Autodesk Fusion 360 part; units mm, degrees
(part 2 of 2)
sketch "Skizze5" plane through (29.2112, 25.4006, 12) normal (0, 0, 1) x (1, 0, 0)
  line L0 (-31.25, 31.4) -> (31.25, 31.4)
  arc A0 (-31.25, 31.4) -> (-34.25, 28.4) centre (-31.25, 28.4) ccw
  line L1 (-34.25, -25.4) -> (-34.25, 28.4)
  line L2 (-32.25, -25.4) -> (-32.25, 28.4)
  arc A1 (-31.25, 29.4) -> (-32.25, 28.4) centre (-31.25, 28.4) ccw
  line L3 (-31.25, 29.4) -> (31.25, 29.4)
  arc A2 (32.25, 28.4) -> (31.25, 29.4) centre (31.25, 28.4) ccw
  line L4 (32.25, 28.4) -> (32.25, -25.4)
  arc A3 (34.25, 28.4) -> (31.25, 31.4) centre (31.25, 28.4) ccw
  line L5 (34.25, 28.4) -> (34.25, -25.4)
  line L6 (34.25, -25.4) -> (-34.25, -25.4)
  line L7 (-32.25, -15.7) -> (32.25, -15.7)
  line L8 (-32.25, -13.7) -> (32.25, -13.7)
  line L9 (-33.05, -25.4) -> (-33.05, 28.4)
  arc A4 (-31.25, 30.2) -> (-33.05, 28.4) centre (-31.25, 28.4) ccw
  line L10 (-31.25, 30.2) -> (31.25, 30.2)
  arc A5 (33.05, 28.4) -> (31.25, 30.2) centre (31.25, 28.4) ccw
  line L11 (33.05, 28.4) -> (33.05, -25.4)
  line L12 (-32.25, -13.4) -> (-30.35, -13.4)
  line L13 (-30.35, -13.4) -> (-30.35, -5.4)
  line L14 (-30.35, -5.4) -> (-32.25, -5.4)
  line L15 (-32.25, -5.4) -> (-32.25, -13.4)
  line L16 (-32.25, 23.4) -> (32.25, 23.4)
  line L17 (-32.25, 23.1) -> (-30.35, 23.1)
  line L18 (-30.35, 23.1) -> (-30.35, 15.1)
  line L19 (-30.35, 15.1) -> (-32.25, 15.1)
  line L20 (-32.25, 15.1) -> (-32.25, 23.1)
  line L21 (32.25, 23.1) -> (30.35, 23.1)
  line L22 (30.35, 23.1) -> (30.35, 15.1)
  line L23 (30.35, 15.1) -> (32.25, 15.1)
  line L24 (32.25, 15.1) -> (32.25, 23.1)
  line L25 (32.25, -13.4) -> (30.35, -13.4)
  line L26 (30.35, -13.4) -> (30.35, -5.4)
  line L27 (30.35, -5.4) -> (32.25, -5.4)
  line L28 (32.25, -5.4) -> (32.25, -13.4)
  circle A6 centre (-19.6088, 18.0696) radius 2.5
  line L29 (-32.25, 6.4) -> (-25.25, 6.4)
  line L30 (-25.25, 6.4) -> (-25.25, 4.4)
  line L31 (-25.25, 4.4) -> (-32.25, 4.4)
  line L32 (-32.25, 4.4) -> (-32.25, 6.4)
  line L33 (32.25, 4.4) -> (25.25, 4.4)
  line L34 (25.25, 4.4) -> (25.25, 6.4)
  line L35 (25.25, 6.4) -> (32.25, 6.4)
  line L36 (32.25, 6.4) -> (32.25, 4.4)
  point P0 (32.25, -13.7)
  point P1 (-19.6088, 18.0696)
  dimension "d77" = 1.2
  dimension "d87" = 8
  dimension "d88" = 1.9
  dimension "d89" = 0.3
  dimension "d90" = 8
  dimension "d91" = 0.3
  dimension "d92" = 1.9
  dimension "d93" = 8
  dimension "d94" = 1.9
  dimension "d95" = 0.3
  dimension "d96" = 1.9
  dimension "d97" = 8
  dimension "d98" = 0.3
  dimension "d108" = 5
  dimension "d215" = 7
  dimension "d216" = 2
  dimension "d218" = 25
  dimension "d219" = 7
  dimension "d220" = 2
  constraint horizontal L12
  constraint vertical L13
  constraint horizontal L14
  constraint vertical L15
  constraint coincident L2 L12.start
  constraint horizontal L17
  constraint vertical L18
  constraint horizontal L19
  constraint vertical L20
  constraint coincident L2 L17.start
  constraint horizontal L21
  constraint vertical L22
  constraint horizontal L23
  constraint vertical L24
  constraint coincident L4 L21.start
  constraint horizontal L25
  constraint vertical L26
  constraint horizontal L27
  constraint vertical L28
  constraint coincident L4 L25.start
  constraint coincident P1 A6.centre
  constraint horizontal L29
  constraint vertical L30
  constraint horizontal L31
  constraint vertical L32
  constraint coincident L2 L29.start
  constraint horizontal L33
  constraint vertical L34
  constraint horizontal L35
  constraint vertical L36
  constraint coincident L4 L33.start
  constraint collinear L29 L35
  measures "d87" distance of L12.start L14.end
  measures "d88" distance of L12.start L12.end
  measures "d89" distance of L8 L12.end
  measures "d90" distance of L17.start L19.end
  measures "d91" distance of L16 L17.end
  measures "d92" distance of L18.end L19.end
  measures "d93" distance of L21.start L23.end
  measures "d94" distance of L21.start L21.end
  measures "d95" distance of L16 L21
  measures "d96" distance of L25.start L25.end
  measures "d97" distance of L25.start L27.end
  measures "d98" vertical distance of L25.end P0
  measures "d108" diameter of A6
  measures "d215" distance of L29.start L29.end
  measures "d216" distance of L29.start L31.end
  measures "d218" distance of L0 L29
  measures "d219" distance of L33.start L33.end
  measures "d220" distance of L33.start L35.end
extrude "Extrusion17" add sketch "Skizze5" against normal blind 2 separate body contours L0 A0 L1 A3 L5 L6 L9 A4 L10 A5 L11 | L2 A1 L3 A2 L4 L6 L9 A4 L10 A5 L11 L15 L20 L24 L28 L32 L36 | L2 L4 L6 L7 | L2 L4 L7 L8 | L2 L4 L8 L12 L13 L14 L16 L17 L18 L19 L21 L22 L23 L25 L26 L27 L29 L30 L31 L33 L34 L35 | L2 L12 L13 L14 L15 | L4 L25 L26 L27 L28 | L2 L29 L30 L31 L32 | L4 L33 L34 L35 L36 | L2 L17 L18 L19 L20 | L4 L21 L22 L23 L24 | L2 A1 L3 A2 L4 L16 | A6 makes body 4
extrude "Extrusion18" add sketch "Skizze5" against normal blind 11.8 contours L0 A0 L1 A3 L5 L6 L9 A4 L10 A5 L11 | L2 L4 L7 L8 bodies 4
extrude "Extrusion19" add sketch "Skizze5" against normal blind 13.4 contours L2 A1 L3 A2 L4 L6 L9 A4 L10 A5 L11 L15 L20 L24 L28 L32 L36 bodies 4
fillet "Abrundung9" radius 3 5 edges at (-5.0388, 26.9006, 12) (-4.1602, 55.9219, 12) (29.2112, 56.8006, 12) (62.5825, 55.9219, 12) (63.4612, 26.9006, 12) on bodies 4
fillet "Abrundung10" radius 1 7 edges at (-3.0388, 4.8506, 10) (-3.0388, 32.7506, 10) (-2.746, 54.5077, 10) (29.2112, 54.8006, 10) (61.1683, 54.5077, 10) (61.4612, 32.7506, 10) (61.4612, 4.8506, 10) on bodies 4
fillet "Abrundung11" radius 1 5 edges at (61.4612, 11.7006, 4.6) (61.1683, 11.7006, 9.7071) (29.2112, 11.7006, 10) (-2.746, 11.7006, 9.7071) (-3.0388, 11.7006, 4.6) on bodies 4
extrude "Extrusion20" add sketch "Skizze5" against normal blind 18 contours L2 L12 L13 L14 L15 | L4 L25 L26 L27 L28 | L2 L17 L18 L19 L20 | L4 L21 L22 L23 L24 bodies 4
fillet "Abrundung12" radius 3 4 edges at (-3.0388, 44.5006, 12) (-3.0388, 16.0006, 12) (61.4612, 16.0006, 12) (61.4612, 44.5006, 12) on bodies 4
sketch "Skizze6" plane through (0, 12.0006, 0) normal (0, -1, 0) x (1, 0, 0)
  line L0 (-1.1388, 9.7141) -> (-2.0388, 9.7141)
  arc A0 (-2.0388, 9.7141) -> (-2.753, 9) centre (-2.0388, 9) ccw
  line L1 (-2.753, 9) -> (-2.753, 0.2)
  line L2 (-2.753, 0.2) -> (-3.0388, 0.2)
  line L3 (-3.0388, 0.2) -> (-3.0388, -1.4)
  line L4 (-3.0388, -1.4) -> (-3.0388, -6)
  line L5 (-3.0388, -6) -> (-1.1388, -6)
  line L6 (-1.1388, -6) -> (-1.1388, 9.7141)
  line L7 (-3.0388, -6) -> (-3.7388, -4.2859)
  line L8 (-3.7388, -4.2859) -> (-3.0388, -4)
  line L9 (-3.0388, -4) -> (-3.0388, -6)
  line L10 (61.4612, -1.4) -> (61.4612, -6)
  line L11 (61.4612, -6) -> (62.1612, -4.2859)
  line L12 (62.1612, -4.2859) -> (61.4612, -4)
  dimension "d102" = 2
  dimension "d103" = 0.7
  dimension "d104" = 2
  dimension "d105" = 0.7
  constraint coincident L4.end L5.start
  constraint coincident L4 L8.end
  constraint perpendicular L7 L8
  constraint coincident L10.end L11.start
  constraint coincident L10 L12.end
  constraint perpendicular L11 L12
  measures "d102" distance of L4.end L8.end
  measures "d103" horizontal distance of L4.end L7.end
  measures "d104" distance of L10.end L12.end
  measures "d105" horizontal distance of L10.end L11.end
extrude "Extrusion21" add sketch "Skizze6" against normal blind 8 separate body contours L4 L7 L8 L9 | L10 L11 L12 makes body 5 at (-3.0388, 17.3339, -4.6667) makes body 6 at (61.4612, 17.3339, -4.6667)
copy_body "Körper kopieren/einfügen1" bodies 6 makes body 7
move_body "Verschieben1" bodies 7 to x (1, 0, 0) y (0, 1, 0) z (0, 0, 1) at (0, 28.5, 0)
copy_body "Körper kopieren/einfügen2" bodies 5 makes body 8
move_body "Verschieben2" bodies 8 to x (1, 0, 0) y (0, 1, 0) z (0, 0, 1) at (0, 28.5, 0)
combine "Kombinieren2" operation add target body 4 tool bodies 5 6 7 8
ref_plane "Arbeitsebene5" through (0, 0, 5) normal (0, 0, 1) x (1, 0, 0)
sketch "Skizze7" plane through (0, 0, 5) normal (0, 0, 1) x (1, 0, 0)
  line L0 (60.4612, 56.8006) -> (-2.0388, 56.8006)
  line L1 (0.2112, 56.8006) -> (58.2112, 56.8006)
  line L2 (58.2112, 56.8006) -> (58.2112, 31.8006)
  line L3 (58.2112, 31.8006) -> (0.2112, 31.8006)
  line L4 (0.2112, 31.8006) -> (0.2112, 56.8006)
  dimension "d110" = 58
  dimension "d111" = 25
  constraint horizontal L1
  constraint vertical L2
  constraint horizontal L3
  constraint vertical L4
  constraint midpoint L0 L1
  measures "d110" distance of L1.start L1.end
  measures "d111" distance of L1.start L3.end
extrude "Extrusion22" cut sketch "Skizze7" along normal blind 7 bodies 4
sketch "Skizze8" plane through (0.2112, 0, 0) normal (1, 0, 0) x (0, 1, 0)
  arc A0 (56.8006, 9) -> (53.8006, 12) centre (53.8006, 9) ccw
  line L0 (53.8006, 12) -> (31.8006, 12)
  line L1 (31.8006, 12) -> (31.8006, 10)
  line L2 (31.8006, 10) -> (53.8006, 10)
  arc A1 (54.8006, 9) -> (53.8006, 10) centre (53.8006, 9) ccw
  line L3 (54.8006, 9) -> (54.8006, 5)
  line L4 (54.8006, 5) -> (56.8006, 5)
  line L5 (56.8006, 5) -> (56.8006, 9)
  line L6 (31.8006, 12) -> (53.8006, 12)
  arc A2 (56.8006, 9) -> (53.8006, 12) centre (53.8006, 9) ccw
  line L7 (56.8006, 9) -> (56.8006, 5)
  line L8 (54.8006, 5) -> (56.8006, 5)
  line L9 (54.8006, 5) -> (54.8006, 9)
  arc A3 (54.8006, 9) -> (53.8006, 10) centre (53.8006, 9) ccw
  line L10 (53.8006, 10) -> (31.8006, 10)
  line L11 (31.8006, 10) -> (31.8006, 12)
  line L12 (55.6006, 5) -> (55.6006, 9)
  arc A4 (55.6006, 9) -> (53.8006, 10.8) centre (53.8006, 9) ccw
  line L13 (53.8006, 10.8) -> (31.8006, 10.8)
  line L14 (54.8006, 8) -> (55.6006, 8)
  dimension "d115" = 0.8
  dimension "d116" = 3
  constraint parallel L9 L12
  constraint concentric A3 A4
  constraint parallel L10 L13
  constraint tangent A4 L13
  constraint tangent L12 A4
  constraint coincident L9 L14.start
  constraint coincident L12 L14.end
  constraint perpendicular L12 L14
  measures "d115" distance of L10 L13
  measures "d116" distance of L3.end L14.start
extrude "Extrusion23" add sketch "Skizze8" along normal blind 1.5 contours L1 L2 A1 L3 L9 A3 L10 L11 L12 A4 L13 L14 bodies 4
sketch "Skizze9" plane through (58.2112, 0, 0) normal (-1, 0, 0) x (0, -1, 0)
  arc A0 (-53.8006, 12) -> (-56.8006, 9) centre (-53.8006, 9) ccw
  line L0 (-56.8006, 9) -> (-56.8006, 5)
  line L1 (-56.8006, 5) -> (-54.8006, 5)
  line L2 (-54.8006, 5) -> (-54.8006, 9)
  arc A1 (-53.8006, 10) -> (-54.8006, 9) centre (-53.8006, 9) ccw
  line L3 (-53.8006, 10) -> (-31.8006, 10)
  line L4 (-31.8006, 10) -> (-31.8006, 12)
  line L5 (-31.8006, 12) -> (-53.8006, 12)
  line L6 (-31.8006, 12) -> (-53.8006, 12)
  arc A2 (-53.8006, 12) -> (-56.8006, 9) centre (-53.8006, 9) ccw
  line L7 (-56.8006, 9) -> (-56.8006, 5)
  line L8 (-54.8006, 5) -> (-56.8006, 5)
  line L9 (-54.8006, 5) -> (-54.8006, 9)
  line L10 (-55.6006, 5) -> (-55.6006, 9)
  line L11 (-54.8006, 8) -> (-55.6006, 8)
  arc A3 (-53.8006, 10.8) -> (-55.6006, 9) centre (-53.8006, 9) ccw
  arc A4 (-53.8006, 10) -> (-54.8006, 9) centre (-53.8006, 9) ccw
  line L12 (-53.8006, 10.8) -> (-31.8006, 10.8)
  line L13 (-53.8006, 10) -> (-31.8006, 10)
  line L14 (-31.8006, 10) -> (-31.8006, 12)
extrude "Extrusion24" add sketch "Skizze9" along normal blind 1.5 contours L2 A1 L3 L4 L9 L10 L11 A3 A4 L12 L13 L14 bodies 4
sketch "Skizze10" plane through (0, 0, 10) normal (0, 0, -1) x (1, 0, 0)
  line L0 (-2.0388, -53.8006) -> (1.7112, -53.8006)
  line L1 (1.7112, -53.8006) -> (1.7112, -31.8006)
  line L2 (1.7112, -31.8006) -> (56.7112, -31.8006)
  line L3 (56.7112, -31.8006) -> (56.7112, -53.8006)
  line L4 (56.7112, -53.8006) -> (60.4612, -53.8006)
  line L5 (60.4612, -53.8006) -> (60.4612, -48.5006)
  line L6 (60.4612, -48.5006) -> (59.5612, -48.5006)
  line L7 (59.5612, -48.5006) -> (59.5612, -40.5006)
  line L8 (59.5612, -40.5006) -> (60.4612, -40.5006)
  line L9 (60.4612, -40.5006) -> (60.4612, -20.0006)
  line L10 (60.4612, -20.0006) -> (59.5612, -20.0006)
  line L11 (59.5612, -20.0006) -> (59.5612, -12.7006)
  line L12 (59.5612, -12.7006) -> (-1.1388, -12.7006)
  line L13 (-1.1388, -12.7006) -> (-1.1388, -20.0006)
  line L14 (-1.1388, -20.0006) -> (-2.0388, -20.0006)
  line L15 (-2.0388, -20.0006) -> (-2.0388, -40.5006)
  line L16 (-2.0388, -40.5006) -> (-1.1388, -40.5006)
  line L17 (-1.1388, -40.5006) -> (-1.1388, -48.5006)
  line L18 (-1.1388, -48.5006) -> (-2.0388, -48.5006)
  line L19 (-2.0388, -48.5006) -> (-2.0388, -53.8006)
  line L20 (1.7112, -31.8006) -> (56.7112, -31.8006)
  line L21 (7.2112, -28.8006) -> (51.2112, -28.8006)
  line L22 (51.2112, -28.8006) -> (51.2112, -31.8006)
  line L23 (51.2112, -31.8006) -> (7.2112, -31.8006)
  line L24 (7.2112, -31.8006) -> (7.2112, -28.8006)
  line L25 (24.2112, -28.8006) -> (34.2112, -28.8006)
  line L26 (34.2112, -28.8006) -> (34.2112, -30.8006)
  line L27 (34.2112, -30.8006) -> (24.2112, -30.8006)
  line L28 (24.2112, -30.8006) -> (24.2112, -28.8006)
  dimension "d121" = 44
  dimension "d122" = 3
  dimension "d123" = 10
  dimension "d124" = 2
  constraint horizontal L21
  constraint vertical L22
  constraint horizontal L23
  constraint vertical L24
  constraint midpoint L2 L23
  constraint horizontal L25
  constraint vertical L26
  constraint horizontal L27
  constraint vertical L28
  constraint midpoint L21 L25
  measures "d121" distance of L21.start L21.end
  measures "d122" distance of L21.start L23.end
  measures "d123" distance of L25.start L25.end
  measures "d124" distance of L25.start L27.end
extrude "Extrusion25" cut sketch "Skizze10" against normal blind 1 contours L2 L20 L21 L22 L23 L24 L26 L27 L28 | L21 L25 L26 L27 L28 bodies 4
extrude "Extrusion26" cut sketch "Skizze10" against normal blind 1.5 contours L21 L25 L26 L27 L28 bodies 4
extrude "Extrusion27" add sketch "Skizze9" along normal blind 58 separate body contours A0 L0 L1 L4 L5 L6 A2 L7 L8 L10 A3 L12 L14 makes body 9
extrude "Extrusion28" add sketch "Skizze9" along normal blind 58 contours L2 A1 L3 L4 L9 L10 L11 A3 A4 L12 L13 L14 | L1 L2 L8 L9 L10 L11 bodies 9
extrude "Extrusion29" cut sketch "Skizze9" along normal blind 0.3 contours A0 L0 L1 L4 L5 L6 A2 L7 L8 L10 A3 L12 L14 | L1 L2 L8 L9 L10 L11 bodies 9
extrude "Extrusion30" cut sketch "Skizze9" along normal blind 1.8 contours L2 A1 L3 L4 L9 L10 L11 A3 A4 L12 L13 L14 bodies 9
extrude "Extrusion31" cut sketch "Skizze8" along normal blind 1.8 contours L1 L2 A1 L3 L9 A3 L10 L11 L12 A4 L13 L14 bodies 9
extrude "Extrusion32" cut sketch "Skizze8" along normal blind 0.3 contours A0 L0 L1 L4 L5 L6 A2 L7 L8 L11 L12 A4 L13 | L3 L4 L8 L9 L12 L14 bodies 9
sketch "Skizze11" plane through (0, 31.8006, 0) normal (0, -1, 0) x (1, 0, 0)
  line L0 (0.5112, 12) -> (0.5112, 10.8)
  line L1 (0.5112, 10.8) -> (2.0112, 10.8)
  line L2 (2.0112, 10.8) -> (2.0112, 10)
  line L3 (2.0112, 10) -> (56.4112, 10)
  line L4 (56.4112, 10) -> (56.4112, 10.8)
  line L5 (56.4112, 10.8) -> (57.9112, 10.8)
  line L6 (57.9112, 10.8) -> (57.9112, 12)
  line L7 (57.9112, 12) -> (0.5112, 12)
  line L8 (51.2112, 11) -> (7.2112, 11)
  line L9 (51.2112, 10) -> (51.2112, 11)
  line L10 (7.2112, 11) -> (7.2112, 10)
  line L11 (7.2112, 10) -> (51.2112, 10)
  line L12 (50.7112, 11) -> (50.7112, 10)
  line L13 (7.7112, 11) -> (7.7112, 10)
  dimension "d141" = 0.5
  dimension "d142" = 0.5
  constraint coincident L8 L12.start
  constraint perpendicular L8 L12
  constraint coincident L11 L12.end
  constraint coincident L8 L13.start
  constraint coincident L3 L13.end
  constraint perpendicular L8 L13
  measures "d141" distance of L8.start L12.start
  measures "d142" distance of L8.end L13.start
extrude "Extrusion33" add sketch "Skizze11" along normal blind 2.7 contours L3 L8 L11 L12 L13 bodies 9
move_face "Flächen versetzen1" offset -0.2 6 faces at (57.4112, 46.4673, 10.8) (1.0112, 46.4673, 10.8) (1.5112, 54.6254, 10.5999) (1.0112, 55.6006, 8.3333) (56.9112, 54.4696, 10.6711) (57.4112, 55.6006, 8.3333) on bodies 9
move_face "Flächen versetzen2" offset -0.2 1 faces at (57.4112, 55.1339, 8) on bodies 9
move_face "Flächen versetzen3" offset -0.2 1 faces at (1.0112, 55.1339, 8) on bodies 9
extrude "Extrusion34" cut sketch "Skizze11" against normal blind 0.5 contours L0 L1 L2 L3 L4 L5 L6 L7 L8 L9 L10 | L3 L8 L10 L11 L13 | L3 L8 L9 L11 L12 bodies 9
sketch "Skizze12" plane through (0, 0, 11) normal (0, 0, 1) x (-1, 0, 0)
  line L0 (-7.7112, -32.3006) -> (-7.7112, -29.1006)
  line L1 (-7.7112, -29.1006) -> (-50.7112, -29.1006)
  line L2 (-50.7112, -29.1006) -> (-50.7112, -32.3006)
  line L3 (-50.7112, -32.3006) -> (-7.7112, -32.3006)
  line L4 (-24.2112, -30.8006) -> (-24.2112, -28.8006)
  line L5 (-34.2112, -30.8006) -> (-24.2112, -30.8006)
  line L6 (-34.2112, -28.8006) -> (-34.2112, -30.8006)
  line L7 (-50.7112, -29.1006) -> (-7.7112, -29.1006)
  line L8 (-24.7112, -30.5006) -> (-24.7112, -29.1006)
  line L9 (-33.7112, -30.5006) -> (-33.7112, -29.1006)
  line L10 (-24.7112, -30.5006) -> (-33.7112, -30.5006)
  dimension "d150" = 0.5
  dimension "d151" = 0.5
  dimension "d152" = 0.3
  constraint coincident L1 L8.end
  constraint perpendicular L1 L8
  constraint coincident L7 L9.end
  constraint perpendicular L7 L9
  constraint perpendicular L9 L10
  measures "d150" distance of L4 L8.end
  measures "d151" distance of L6 L9.end
  measures "d152" distance of L5 L10
extrude "Extrusion35" add sketch "Skizze12" along normal blind 0.5 contours L1 L7 L8 L9 L10 bodies 9
fillet "Abrundung13" radius 0.4 2 edges at (29.2112, 30.5006, 11.5) (29.2112, 29.1006, 11.5) on bodies 9
sketch "Skizze13" plane through (0, 54.8006, 0) normal (0, -1, 0) x (1, 0, 0)
  line L0 (0.5112, 7.8) -> (0.5112, 5)
  line L1 (0.5112, 5) -> (57.9112, 5)
  line L2 (57.9112, 5) -> (57.9112, 7.8)
  line L3 (57.9112, 7.8) -> (56.4112, 7.8)
  line L4 (56.4112, 7.8) -> (56.4112, 9)
  line L5 (56.4112, 9) -> (2.0112, 9)
  line L6 (2.0112, 9) -> (2.0112, 7.8)
  line L7 (2.0112, 7.8) -> (0.5112, 7.8)
  line L8 (2.0112, 7.8) -> (0.5112, 7.8)
  line L9 (0.5112, 7.8) -> (0.5112, 5)
  line L10 (57.9112, 5) -> (0.5112, 5)
  line L11 (57.9112, 7.8) -> (56.4112, 7.8)
  line L12 (57.9112, 5) -> (57.9112, 7.8)
  line L13 (2.0112, 7.8) -> (2.0112, 5)
  line L14 (56.4112, 7.8) -> (56.4112, 5)
  constraint coincident L6.end L7.start
  constraint coincident L10 L13.end
  constraint perpendicular L10 L13
  constraint coincident L3.end L4.start
  constraint coincident L1 L14.end
  constraint perpendicular L1 L14
extrude "Extrusion36" add sketch "Skizze13" along normal blind 2 contours L0 L1 L7 L8 L9 L10 L13 | L1 L2 L3 L10 L11 L12 L14 bodies 9
chamfer "Fase1" distance 0.5 distance2 1 2 edges at (1.2612, 52.8006, 7.8) (57.1612, 52.8006, 7.8) measured on face at (1.0112, 52.8006, 5.9333) measured on face at (57.4112, 52.8006, 5.9333) on bodies 9
sketch "Skizze14" plane through (0, 54.8006, 0) normal (0, -1, 0) x (1, 0, 0)
  line L0 (0.2112, 5) -> (0.2112, 8)
  line L1 (0.2112, 8) -> (1.7112, 8)
  line L2 (1.7112, 8) -> (1.7112, 9)
  line L3 (1.7112, 9) -> (-2.0388, 9)
  line L4 (-2.0388, 9) -> (-2.0388, -1.4)
  line L5 (-2.0388, -1.4) -> (60.4612, -1.4)
  line L6 (60.4612, -1.4) -> (60.4612, 9)
  line L7 (60.4612, 9) -> (56.7112, 9)
  line L8 (56.7112, 9) -> (56.7112, 8)
  line L9 (56.7112, 8) -> (58.2112, 8)
  line L10 (58.2112, 8) -> (58.2112, 5)
  line L11 (58.2112, 5) -> (0.2112, 5)
  line L12 (2.0112, 5) -> (2.0112, 7.3)
  line L13 (56.4112, 7.3) -> (56.4112, 5)
  line L14 (56.4112, 5) -> (2.0112, 5)
  line L15 (3.0112, 6.5) -> (55.4112, 6.5)
  line L16 (55.4112, 6.5) -> (55.4112, 3)
  line L17 (55.4112, 3) -> (3.0112, 3)
  line L18 (3.0112, 3) -> (3.0112, 6.5)
  dimension "d160" = 1
  dimension "d161" = 1
  dimension "d162" = 2
  dimension "d163" = 1.5
  constraint horizontal L15
  constraint vertical L16
  constraint horizontal L17
  constraint vertical L18
  measures "d160" horizontal distance of L12.end L15.start
  measures "d161" distance of L13 L16
  measures "d162" distance of L14 L17
  measures "d163" distance of L14 L15
extrude "Extrusion37" add sketch "Skizze14" along normal blind 1.5 contours L11 L14 L15 L16 L18 | L11 L14 L16 L17 L18 bodies 4
fillet "Abrundung14" radius 1 1 edges at (29.2112, 54.8006, 3) on bodies 4
sketch "Skizze15" plane through (0, 0, 10) normal (0, 0, -1) x (1, 0, 0)
  line L0 (56.4112, -32.3006) -> (50.7112, -32.3006)
  line L1 (50.7112, -32.3006) -> (50.7112, -29.1006)
  line L2 (50.7112, -29.1006) -> (7.7112, -29.1006)
  line L3 (7.7112, -29.1006) -> (7.7112, -32.3006)
  line L4 (7.7112, -32.3006) -> (2.0112, -32.3006)
  line L5 (2.0112, -32.3006) -> (2.0112, -53.8006)
  line L6 (2.0112, -53.8006) -> (56.4112, -53.8006)
  line L7 (56.4112, -53.8006) -> (56.4112, -32.3006)
  circle A0 centre (9.6024, -43.4702) radius 2.5
  circle A1 centre (9.6024, -43.4702) radius 2.25
  line L8 (12.6024, -46.9702) -> (6.6024, -46.9702)
  line L9 (6.1024, -46.4702) -> (6.1024, -40.4702)
  line L10 (6.6024, -39.9702) -> (12.6024, -39.9702)
  line L11 (13.1024, -40.4702) -> (13.1024, -46.4702)
  line L12 (13.1024, -46.9702) -> (6.1024, -39.9702) construction
  line L13 (6.1024, -46.9702) -> (13.1024, -39.9702) construction
  line L14 (6.8024, -39.6702) -> (6.3024, -39.6702)
  line L15 (4.3024, -39.9702) -> (4.3024, -38.1702)
  line L16 (4.3024, -38.1702) -> (6.8024, -38.1702)
  line L17 (6.8024, -38.1702) -> (6.8024, -39.6702)
  line L18 (5.8024, -40.1702) -> (5.8024, -40.6702)
  line L19 (5.8024, -40.6702) -> (4.3024, -40.6702)
  line L20 (4.3024, -40.6702) -> (4.3024, -39.9702)
  line L21 (12.4024, -39.6702) -> (12.9024, -39.6702)
  line L22 (14.9024, -40.0702) -> (14.9024, -38.1702)
  line L23 (14.9024, -38.1702) -> (12.4024, -38.1702)
  line L24 (12.4024, -38.1702) -> (12.4024, -39.6702)
  line L25 (13.4024, -40.1702) -> (13.4024, -40.6702)
  line L26 (13.4024, -40.6702) -> (14.9024, -40.6702)
  line L27 (14.9024, -40.6702) -> (14.9024, -40.0702)
  line L28 (13.4024, -46.2702) -> (14.9024, -46.2702)
  line L29 (14.9024, -46.2702) -> (14.9024, -46.8939)
  line L30 (13.4024, -46.7702) -> (13.4024, -46.2702)
  line L31 (12.9024, -47.2702) -> (12.4024, -47.2702)
  line L32 (12.4024, -47.2702) -> (12.4024, -48.7702)
  line L33 (12.4024, -48.7702) -> (14.9024, -48.7702)
  line L34 (14.9024, -48.7702) -> (14.9024, -46.8939)
  line L35 (6.8024, -47.2702) -> (6.3024, -47.2702)
  line L36 (4.3024, -46.9702) -> (4.3024, -48.7702)
  line L37 (4.3024, -48.7702) -> (6.8024, -48.7702)
  line L38 (6.8024, -48.7702) -> (6.8024, -47.2702)
  line L39 (5.8024, -46.7702) -> (5.8024, -46.2702)
  line L40 (5.8024, -46.2702) -> (4.3024, -46.2702)
  line L41 (4.3024, -46.2702) -> (4.3024, -46.9702)
  arc A2 (6.6024, -39.9702) -> (6.1024, -40.4702) centre (6.6024, -40.4702) ccw
  arc A3 (13.1024, -40.4702) -> (12.6024, -39.9702) centre (12.6024, -40.4702) ccw
  arc A4 (12.6024, -46.9702) -> (13.1024, -46.4702) centre (12.6024, -46.4702) ccw
  arc A5 (6.1024, -46.4702) -> (6.6024, -46.9702) centre (6.6024, -46.4702) ccw
  line L42 (7.3024, -38.1702) -> (11.9024, -38.1702)
  line L43 (11.9024, -38.1702) -> (11.9024, -39.6702)
  line L44 (11.9024, -39.6702) -> (7.3024, -39.6702)
  line L45 (7.3024, -39.6702) -> (7.3024, -38.1702)
  line L46 (7.3024, -47.2702) -> (11.9024, -47.2702)
  line L47 (11.9024, -47.2702) -> (11.9024, -48.7702)
  line L48 (11.9024, -48.7702) -> (7.3024, -48.7702)
  line L49 (7.3024, -48.7702) -> (7.3024, -47.2702)
  line L50 (6.8024, -39.9702) -> (6.8024, -40.7702)
  line L51 (6.8024, -40.7702) -> (12.4024, -40.7702)
  line L52 (12.4024, -40.7702) -> (12.4024, -39.9702)
  line L53 (6.8024, -46.9702) -> (6.8024, -46.1702)
  line L54 (6.8024, -46.1702) -> (12.4024, -46.1702)
  line L55 (12.4024, -46.1702) -> (12.4024, -46.9702)
  line L56 (4.3024, -46.2702) -> (4.3024, -40.6702)
  line L57 (5.8024, -46.2702) -> (5.8024, -40.6702)
  line L58 (13.4024, -46.2702) -> (13.4024, -40.6702)
  line L59 (14.9024, -46.2702) -> (14.9024, -40.6702)
  arc A6 (12.9024, -47.2702) -> (13.4024, -46.7702) centre (12.9024, -46.7702) ccw
  arc A7 (13.4024, -40.1702) -> (12.9024, -39.6702) centre (12.9024, -40.1702) ccw
  arc A8 (6.3024, -39.6702) -> (5.8024, -40.1702) centre (6.3024, -40.1702) ccw
  arc A9 (5.8024, -46.7702) -> (6.3024, -47.2702) centre (6.3024, -46.7702) ccw
  point P0 (9.6024, -43.4702)
  point P1 (9.6024, -43.4702)
  dimension "d167" = 5
  dimension "d168" = 4.5
  dimension "d169" = 7
  dimension "d170" = 7
  dimension "d171" = 0.3
  dimension "d172" = 0.3
  dimension "d173" = 1.5
  dimension "d174" = 1.5
  dimension "d175" = 2.5
  dimension "d176" = 2.5
  dimension "d177" = 2.5
  dimension "d178" = 0.3
  dimension "d179" = 1.5
  dimension "d180" = 2.5
  dimension "d181" = 2.5
  dimension "d182" = 0.3
  dimension "d183" = 1.5
  dimension "d184" = 2.5
  dimension "d185" = 2.5
  dimension "d186" = 2.5
  dimension "d187" = 0.5
  dimension "d188" = 0.5
  dimension "d189" = 0.5
  dimension "d190" = 0.5
  dimension "d191" = 0.5
  dimension "d193" = 0.5
  dimension "d194" = 0.8
  dimension "d195" = 0.8
  dimension "d253" = 0.5
  dimension "d254" = 0.5
  dimension "d255" = 0.5
  dimension "d256" = 0.5
  constraint coincident P1 P0
  constraint perpendicular L8 L9
  constraint parallel L8 L10
  constraint parallel L9 L11
  constraint horizontal L8
  constraint coincident L12 P1
  constraint coincident L13 P1
  constraint horizontal L14
  constraint vertical L15
  constraint horizontal L16
  constraint vertical L17
  constraint vertical L18
  constraint horizontal L19
  constraint vertical L20
  constraint horizontal L21
  constraint vertical L22
  constraint horizontal L23
  constraint vertical L24
  constraint vertical L25
  constraint horizontal L26
  constraint vertical L27
  constraint collinear L16 L23
  constraint collinear L14 L21
  constraint horizontal L28
  constraint vertical L29
  constraint vertical L30
  constraint horizontal L31
  constraint vertical L32
  constraint horizontal L33
  constraint vertical L34
  constraint collinear L22 L29
  constraint collinear L25 L30
  constraint horizontal L35
  constraint vertical L36
  constraint horizontal L37
  constraint vertical L38
  constraint vertical L39
  constraint horizontal L40
  constraint vertical L41
  constraint collinear L15 L41
  constraint collinear L18 L39
  constraint collinear L31 L35
  constraint collinear L33 L37
  constraint coincident L12.end L9
  constraint coincident L12.end L10
  constraint tangent L9 A2
  constraint tangent L10 A2
  constraint coincident L13.end L10
  constraint coincident L13.end L11
  constraint tangent L10 A3
  constraint tangent L11 A3
  constraint coincident L12.start L11
  constraint coincident L12.start L8
  constraint tangent L11 A4
  constraint tangent L8 A4
  constraint coincident L13.start L8
  constraint coincident L13.start L9
  constraint tangent L8 A5
  constraint tangent L9 A5
  constraint horizontal L42
  constraint vertical L43
  constraint horizontal L44
  constraint vertical L45
  constraint collinear L23 L42
  constraint collinear L21 L44
  constraint horizontal L46
  constraint vertical L47
  constraint horizontal L48
  constraint vertical L49
  constraint collinear L35 L46
  constraint collinear L37 L48
  constraint collinear L45 L49
  constraint collinear L43 L47
  constraint coincident L10 L50.start
  constraint perpendicular L10 L50
  constraint perpendicular L43 L51
  constraint coincident L10 L52.end
  constraint perpendicular L10 L52
  constraint collinear L17 L50
  constraint collinear L24 L52
  constraint coincident L8 L53.start
  constraint perpendicular L8 L53
  constraint perpendicular L32 L54
  constraint coincident L8 L55.end
  constraint perpendicular L8 L55
  constraint collinear L38 L53
  constraint collinear L32 L55
  constraint tangent L30 A6
  constraint tangent L31 A6
  constraint tangent L25 A7
  constraint tangent L21 A7
  constraint tangent L18 A8
  constraint tangent L14 A8
  constraint tangent L39 A9
  constraint tangent L35 A9
  measures "d167" diameter of A0
  measures "d168" diameter of A1
  measures "d169" distance of L12.end L13.end
  measures "d170" distance of L13.start L12.end
  measures "d171" distance of L10 L14.start
  measures "d172" distance of L9 L18.end
  measures "d173" distance of L14 L16
  measures "d174" distance of L18 L20
  measures "d175" distance of L15.end L17
  measures "d176" distance of L15.end L19
  measures "d177" distance of L22.end L23.end
  measures "d178" distance of L11 L25
  measures "d179" distance of L25 L27
  measures "d180" distance of L22.end L26
  measures "d181" distance of L28.end L33.end
  measures "d182" distance of L8 L31
  measures "d183" distance of L31 L33
  measures "d184" distance of L32.end L33.end
  measures "d185" distance of L36.end L37.end
  measures "d186" distance of L36.end L40.end
  measures "d187" radius of A2
  measures "d188" radius of A3
  measures "d189" radius of A4
  measures "d190" radius of A5
  measures "d191" distance of L17 L45
  measures "d193" distance of L24 L43
  measures "d194" distance of L10 L51
  measures "d195" distance of L8 L54
  measures "d253" radius of A6
  measures "d254" radius of A7
  measures "d255" radius of A8
  measures "d256" radius of A9
extrude "Extrusion38" cut sketch "Skizze15" against normal blind 2 contours A0 | A1 bodies 9
extrude "Extrusion39" add sketch "Skizze15" against normal blind 2.5 separate body contours A1 makes body 10
extrude "Extrusion41" add sketch "Skizze15" 1 faces at (9.2274, 44.7706, 10) along normal blind 0.7 contours A0 | A1 | L8 L9 L10 L11 A2 A3 A4 A5 L50 L51 L52 L53 L54 L55 | L8 L53 L54 L55 | L10 L50 L51 L52 on bodies 10 bodies 10
extrude "Extrusion42" add sketch "Skizze15" along normal blind 2.5 contours A0 | A1 | L8 L9 L10 L11 A2 A3 A4 A5 L50 L51 L52 L53 L54 L55 bodies 10
extrude "Extrusion43" add sketch "Skizze15" along normal blind 2.5 contours L14 L15 L16 L17 L18 L19 L20 A8 | L35 L36 L37 L38 L39 L40 L41 A9 | L21 L22 L23 L24 L25 L26 L27 A7 | L28 L29 L30 L31 L32 L33 L34 A6 | L42 L43 L44 L45 | L46 L47 L48 L49 bodies 9
sketch "Skizze16" plane through (7.3024, 0, 0) normal (-1, 0, 0) x (0, -1, 0)
  line L0 (-38.1702, 10) -> (-39.6702, 10)
  line L1 (-39.6702, 10) -> (-39.6702, 7.5)
  line L2 (-39.6702, 7.5) -> (-38.1702, 7.5)
  line L3 (-38.1702, 7.5) -> (-38.1702, 10)
  line L4 (-47.2702, 7.5) -> (-48.7702, 7.5)
  line L5 (-47.2702, 10) -> (-47.2702, 7.5)
  line L6 (-38.1702, 7.5) -> (-39.6702, 7.5)
  line L7 (-39.6702, 10) -> (-39.6702, 7.5)
  line L8 (-40.7702, 9.3) -> (-39.9702, 9.3)
  line L9 (-46.9702, 9.3) -> (-46.1702, 9.3)
  line L10 (-39.6702, 8.75) -> (-39.6702, 7.5)
  line L11 (-39.6702, 8.6) -> (-40.2702, 8.6)
  line L12 (-40.2702, 8.6) -> (-39.6702, 7.5)
  line L13 (-39.6702, 8.6) -> (-39.6702, 7.5)
  line L14 (-47.2702, 8.6) -> (-46.6702, 8.6)
  line L15 (-46.6702, 8.6) -> (-47.2702, 7.5)
  line L16 (-47.2702, 8.6) -> (-47.2702, 7.5)
  dimension "d209" = 0.7
  dimension "d210" = 0.6
  dimension "d211" = 0.6
  constraint midpoint L7 L10.start
  constraint coincident L1.end L2.start
  constraint coincident L10 L11.start
  constraint perpendicular L10 L11
  constraint coincident L5 L14.start
  constraint perpendicular L5 L14
  constraint coincident L4.start L5.end
  constraint collinear L11 L14
  measures "d209" distance of L8 L11
  measures "d210" distance of L11.start L11.end
  measures "d211" distance of L14.end L16
extrude "Extrusion44" add sketch "Skizze16" against normal blind 2.6 contours L1 L7 L10 L11 L12 L13 | L5 L14 L15 L16 bodies 9
fillet "Abrundung15" radius 1 10 edges at (4.3024, 47.5202, 10) (4.3024, 39.4202, 10) (5.5524, 38.1702, 10) (9.6024, 38.1702, 10) (13.6524, 38.1702, 10) (14.9024, 39.4202, 10) (14.9024, 47.5202, 10) (5.5524, 48.7702, 10) (9.6024, 48.7702, 10) (13.6524, 48.7702, 10) on bodies 9
extrude "Extrusion45" add sketch "Skizze5" against normal blind 11.7 contours L2 L29 L30 L31 L32 | L4 L33 L34 L35 L36 bodies 4
fillet "Abrundung16" radius 3 2 edges at (3.9612, 30.8006, 0.3) (54.4612, 30.8006, 0.3) on bodies 4
sketch "Skizze17" plane through (61.4612, 0, 0) normal (-1, 0, 0) x (0, -1, 0)
  line L0 (-48.8006, -7) -> (-11.7006, -7)
  line L1 (-11.7006, -7) -> (-11.7006, -1.6)
  line L2 (-11.7006, -1.6) -> (-48.8006, -1.6)
  line L3 (-48.8006, -1.6) -> (-48.8006, -7)
  line L4 (-12.0006, -1.4) -> (-12.0006, -4)
  line L5 (-12.0006, -4.2859) -> (-12.0006, -4)
  line L6 (-12.0006, -6) -> (-12.0006, -4.2859)
  line L7 (-20.0006, -4.2859) -> (-20.0006, -6)
  line L8 (-20.0006, -4) -> (-20.0006, -4.2859)
  line L9 (-20.0006, -1.4) -> (-20.0006, -4)
  line L10 (-20.0006, -6) -> (-12.0006, -6)
  line L11 (-12.0006, -1.4) -> (-20.0006, -1.4)
  line L12 (-40.5006, -1.4) -> (-48.5006, -1.4)
  line L13 (-48.5006, -1.4) -> (-48.5006, -4)
  line L14 (-48.5006, -4) -> (-48.5006, -4.2859)
  line L15 (-48.5006, -4.2859) -> (-48.5006, -6)
  line L16 (-48.5006, -6) -> (-40.5006, -6)
  line L17 (-40.5006, -6) -> (-40.5006, -4.2859)
  line L18 (-40.5006, -1.4) -> (-40.5006, -4)
  line L19 (-40.5006, -4.2859) -> (-40.5006, -4)
  line L20 (-40.5006, -4) -> (-48.5006, -4)
  line L21 (-12.0006, -4) -> (-20.0006, -4)
  line L22 (-40.3006, -1.4) -> (-40.3006, -4)
  line L23 (-40.3006, -4.2859) -> (-40.3006, -4)
  line L24 (-40.3006, -6.2) -> (-40.3006, -4.2859)
  line L25 (-48.7006, -6.2) -> (-40.3006, -6.2)
  line L26 (-48.7006, -4.2859) -> (-48.7006, -6.2)
  line L27 (-48.7006, -4) -> (-48.7006, -4.2859)
  line L28 (-48.7006, -1.4) -> (-48.7006, -4)
  line L29 (-40.5006, -1.4) -> (-40.3006, -1.4)
  line L30 (-48.5006, -1.4) -> (-48.7006, -1.4)
  line L31 (-40.5006, -3.8) -> (-48.5006, -3.8)
  line L32 (-40.5006, -3.8) -> (-40.3006, -3.8)
  line L33 (-48.5006, -3.8) -> (-48.7006, -3.8)
  line L34 (-44.5006, -6.2) -> (-44.5006, -3.8)
  line L35 (-20.2006, -4) -> (-20.2006, -4.2859)
  line L36 (-20.2006, -4.2859) -> (-20.2006, -6.2)
  line L37 (-20.2006, -6.2) -> (-11.8006, -6.2)
  line L38 (-11.8006, -6.2) -> (-11.8006, -4.2859)
  line L39 (-11.8006, -4.2859) -> (-11.8006, -4)
  line L40 (-11.8006, -1.4) -> (-11.8006, -4)
  line L41 (-20.2006, -1.4) -> (-20.2006, -4)
  line L42 (-20.0006, -1.4) -> (-20.2006, -1.4)
  line L43 (-11.8006, -1.4) -> (-12.0006, -1.4)
  line L44 (-20.2006, -3.8) -> (-11.8006, -3.8)
  line L45 (-16.0006, -6) -> (-16.0006, -4)
  circle A0 centre (-16.0006, -5) radius 0.75
  circle A1 centre (-44.5006, -5) radius 0.75
  point P0 (-12.0006, -4.2859)
  point P1 (-12.0006, -4)
  dimension "d225" = 0.2
  dimension "d226" = 0.2
  dimension "d227" = 0.2
  dimension "d229" = 0.2
  dimension "d230" = 0.2
  dimension "d231" = 0.2
  dimension "d232" = 0.2
  dimension "d233" = 1.5
  dimension "d234" = 1.5
  constraint parallel L18 L22
  constraint parallel L19 L23
  constraint parallel L17 L24
  constraint parallel L16 L25
  constraint parallel L15 L26
  constraint parallel L14 L27
  constraint parallel L13 L28
  constraint coincident L12.start L18.start
  constraint coincident L22 L29.end
  constraint perpendicular L22 L29
  constraint coincident L12.end L13.start
  constraint coincident L28 L30.end
  constraint perpendicular L28 L30
  constraint coincident L22 L32.end
  constraint perpendicular L22 L32
  constraint coincident L28 L33.end
  constraint perpendicular L28 L33
  constraint midpoint L25 L34.start
  constraint midpoint L31 L34.end
  constraint perpendicular L31 L34
  constraint coincident L9.start L11.end
  constraint perpendicular L41 L42
  constraint coincident L4.start L11.start
  constraint perpendicular L4 L43
  constraint parallel L8 L35
  constraint parallel L7 L36
  constraint parallel L10 L37
  constraint parallel L6 L38
  constraint parallel L5 L39
  constraint parallel L4 L40
  constraint parallel L9 L41
  constraint coincident L41 L44.start
  constraint coincident L40 L44.end
  constraint perpendicular L40 L44
  constraint midpoint L10 L45.start
  constraint midpoint L21 L45.end
  constraint midpoint L45 A0.centre
  constraint midpoint L34 A1.centre
  measures "d226" distance of L16 L25
  measures "d227" distance of L17 L24
  measures "d229" distance of L10 L37
  measures "d230" distance of L6 L38
  measures "d231" distance of L7 L36
  measures "d232" distance of L21 L44
  measures "d233" diameter of A0
  measures "d234" diameter of A1
sketch "Skizze19" plane through (-3.0388, 0, 0) normal (1, 0, 0) x (0, 1, 0)
  line L0 (29.8006, 0.3) -> (29.8006, 9)
  line L1 (29.8006, 9) -> (20.0006, 9)
  line L2 (20.0006, 9) -> (20.0006, -1.4)
  line L3 (20.0006, -1.4) -> (40.5006, -1.4)
  line L4 (40.5006, -1.4) -> (40.5006, 9)
  line L5 (40.5006, 9) -> (31.8006, 9)
  line L6 (31.8006, 9) -> (31.8006, 0.3)
  line L7 (31.8006, 0.3) -> (29.8006, 0.3)
  line L8 (48.7006, -6.2) -> (40.3006, -6.2)
  line L9 (40.3006, -6.2) -> (40.3006, -4.2859)
  line L10 (40.5006, -3.8) -> (48.5006, -3.8)
  line L11 (40.5006, -3.8) -> (40.3006, -3.8)
  line L12 (40.3006, -1.4) -> (40.3006, -4)
  line L13 (40.3006, -4.2859) -> (40.3006, -4)
  line L14 (40.5006, -1.4) -> (48.5006, -1.4)
  circle A0 centre (44.5006, -5) radius 0.75
  line L15 (48.7006, -4.2859) -> (48.7006, -6.2)
  line L16 (48.7006, -4) -> (48.7006, -4.2859)
  line L17 (48.7006, -1.4) -> (48.7006, -4)
  line L18 (48.5006, -3.8) -> (48.7006, -3.8)
  line L19 (11.8006, -1.4) -> (11.8006, -4)
  line L20 (20.2006, -3.8) -> (11.8006, -3.8)
  line L21 (11.8006, -6.2) -> (11.8006, -4.2859)
  line L22 (11.8006, -4.2859) -> (11.8006, -4)
  line L23 (20.2006, -6.2) -> (11.8006, -6.2)
  line L24 (20.2006, -4.2859) -> (20.2006, -6.2)
  line L25 (20.2006, -4) -> (20.2006, -4.2859)
  line L26 (20.2006, -1.4) -> (20.2006, -4)
  line L27 (12.0006, -1.4) -> (20.0006, -1.4)
  circle A1 centre (16.0006, -5) radius 0.75
  line L28 (40.5006, -1.4) -> (40.3006, -1.4)
  line L29 (48.5006, -1.4) -> (48.7006, -1.4)
  line L30 (20.0006, -1.4) -> (20.2006, -1.4)
  line L31 (12.0006, -1.4) -> (11.8006, -1.4)
  constraint coincident L2.end L3.start
  constraint coincident L26.start L30.end
  constraint coincident L27.start L31.start
  constraint coincident L19.start L31.end
extrude "Extrusion46" cut sketch "Skizze19" against normal blind 0.2 contours L3 L19 L20 L26 L27 L30 L31 | L3 L10 L11 L12 L14 L17 L18 L28 L29 bodies 3
extrude "Extrusion47" cut sketch "Skizze17" against normal blind 0.2 contours L2 L13 L28 L33 | L2 L4 L40 L44 | L2 L13 L18 L31 | L2 L4 L9 L44 | L2 L18 L22 L32 | L2 L9 L41 L44 bodies 3
extrude "Extrusion48" cut sketch "Skizze17" against normal blind 2 contours L34 A1 | L34 A1 | L45 A0 | L45 A0 bodies 3
extrude "Extrusion49" cut sketch "Skizze17" against normal blind 1 contours L13 L14 L15 L16 L25 L26 L27 L28 L33 L34 | L4 L5 L6 L7 L8 L9 L10 L35 L36 L37 L38 L39 L40 L41 L44 | L13 L20 L31 L34 | L4 L9 L21 L44 | L16 L17 L18 L19 L22 L23 L24 L25 L32 L34 | L18 L20 L31 L34 | L14 L15 L16 L20 L34 A1 | L5 L6 L10 L21 L45 A0 | L16 L17 L19 L20 L34 A1 | L7 L8 L10 L21 L45 A0 bodies 3
extrude "Extrusion50" cut sketch "Skizze19" against normal blind 2 contours A0 | A1 bodies 3
extrude "Extrusion51" cut sketch "Skizze19" against normal blind 1 contours L19 L20 L21 L22 L23 L24 L25 L26 | L8 L9 L10 L11 L12 L13 L15 L16 L17 L18 bodies 3
fillet "Abrundung17" radius 3 1 edges at (61.4612, 30.8006, 12) on bodies 4
fillet "Abrundung18" radius 3 1 edges at (-3.0388, 30.8006, 12) on bodies 4
copy_body "Körper kopieren/einfügen3" bodies 10 makes body 11
move_body "Verschieben3" bodies 11 to x (1, 0, 0) y (0, 1, 0) z (0, 0, 1) at (0, 30, 0)
copy_body "Körper kopieren/einfügen4" bodies 11 makes body 12
move_body "Verschieben4" bodies 12 to x (1, 0, 0) y (0, 1, 0) z (0, 0, 1) at (10, 0, 0)
extrude "Extrusion52" add 1 faces at (10.5357, 74.3702, 7.5) along direction (0, 0, -1) blind 2 on bodies 11 bodies 11
extrude "Extrusion53" add 1 faces at (20.5357, 74.3702, 7.5) along direction (0, 0, -1) blind 2.7 on bodies 12 bodies 12
extrude "Extrusion54" add sketch "Skizze16" against normal blind 4.6 contours L1 L7 L10 L11 L12 L13 | L5 L14 L15 L16 bodies 9
extrude "Extrusion55" add sketch "Skizze15" along normal blind 2.5 contours L19 L40 L56 L57 | L26 L28 L58 L59 bodies 9
fillet "Abrundung19" radius 1 1 edges at (14.9024, 43.4702, 10) on bodies 9
fillet "Abrundung20" radius 1 1 edges at (4.3024, 43.4702, 10) on bodies 9
move_face "Flächen versetzen4" offset -0.2 1 faces at (27.7112, 29.1006, 10.3333) on bodies 9
move_face "Flächen versetzen5" offset -0.2 1 faces at (20.1445, 56.1339, 5) on bodies 9
extrude "Extrusion56" add 1 faces at (9.2274, 44.7706, 12.5) along direction (0, 0, 1) blind 0.5 on bodies 10 bodies 10
fillet "Abrundung21" radius 0.5 2 edges at (9.6024, 40.7702, 7.5) (9.6024, 46.1702, 7.5) on bodies 10
fillet "Abrundung22" radius 0.5 2 edges at (19.6024, 70.7702, 4.8) (19.6024, 76.1702, 4.8) on bodies 12
fillet "Abrundung23" radius 0.5 2 edges at (9.6024, 76.1702, 5.5) (9.6024, 70.7702, 5.5) on bodies 11
move_face "Flächen versetzen6" offset 0.5 1 faces at (9.2274, 74.7706, 12.5) on bodies 11
move_face "Flächen versetzen7" offset 0.5 1 faces at (19.9774, 74.7706, 12.5) on bodies 12
move_face "Flächen versetzen8" offset -0.2 1 faces at (61.4612, 11.0339, -1.0667) on bodies 3
move_face "Flächen versetzen9" offset -0.2 1 faces at (-3.0388, 10.3673, -1.0667) on bodies 3
copy_body "Körper->Berechn1" bodies 1 removing the originals makes body 13 in component "openC64cart"
copy_body "Körper->Berechn2" bodies 3 removing the originals makes body 14 in component "bottom shell"
copy_body "Körper->Berechn3" bodies 4 removing the originals makes body 15 in component "top shell"
copy_body "Körper->Berechn4" bodies 9 removing the originals makes body 16 in component "lid"
copy_body "Körper->Berechn5" bodies 10 removing the originals makes body 17 in component "plunger 7mm"
component "openC64cart" placed x (1, 0, 0) y (0, 1, 0) z (0, 0, 1) at (0, 0, 0)
component "bottom shell" placed x (1, 0, 0) y (0, 1, 0) z (0, 0, 1) at (0, 0, 0)
component "top shell" placed x (1, 0, 0) y (0, 1, 0) z (0, 0, 1) at (0, 0, 0)
component "lid" placed x (1, 0, 0) y (0, 1, 0) z (0, 0, 1) at (0, 0, 0)
component "plunger 7mm" placed x (1, 0, 0) y (0, 1, 0) z (0, 0, 1) at (0, 0, 0)
hidden bodies 11 12
equation "d172 = d171"
equation "d174 = d173"
equation "d176 = d175"
equation "d177 = d175"
equation "d178 = d171"
equation "d179 = d173"
equation "d180 = d175"
equation "d181 = d175"
equation "d182 = d171"
equation "d183 = d173"
equation "d184 = d175"
equation "d185 = d175"
equation "d186 = d175"
equation "d193 = d191"
equation "d195 = d194"
equation "d211 = d210"
equation "d225 = d226"
equation "d227 = d226"
equation "d230 = d229"
equation "d231 = d229"
equation "d232 = d229"
named bodies: "openC64cart", "bottom shell", "top shell", "lid", "plunger 7mm", "plunger 5mm", "plunger 4.3mm"
